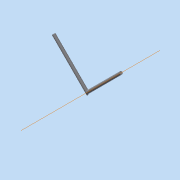
# Autodesk Inventor part: 00_Beampath_Autofocus
Saved by Autodesk Inventor 2019.4 (Build 234330000, 330)
## iProperties
Created: 2020-11-30
Part Number: 00_Beampath_Autofocus
Material: Generic
Document SubType Name: Modeling
Designer: diederichbenedict
Density: 1 g/cm^3
Appearance: Default
Author: diederichbenedict
Autodesk Inventor part; units mm, degrees
ref_plane "XY Plane" through (0, 0, 0) normal (0, 0, 1) x (1, 0, 0)
sketch "Sketch1" plane through (0, 0, 0) normal (0, 0, 1) x (1, 0, 0)
  line L0 (-5.1181, -14.425) -> (0.7509, -8.556) projected
  line L1 (-1.7947, -5.4447) -> (-0.1684, -7.0711) projected
  line L2 (0, 0) -> (12.9271, 0)
  line L3 (0, 0) -> (12.9271, 0) construction
  line L4 (-24, 24) -> (0, 0)
  line L5 (0, 0) -> (24, 24)
  line L6 (0, -22.11) -> (0, 31.685) projected
  dimension "d3" = 0
  dimension "d18" = 45
  dimension "d19" = 45
  dimension "d20" = 24
  dimension "d21" = 24
  constraints: 8 end point, 1 collinear, 1 horizontal
  measures "d3" distance between parallel lines of L2 L3
  measures "d18" angle of L6 L4
  measures "d19" angle of L5 L6
  measures "d20" horizontal distance of L2.start L4.start
  measures "d21" distance from line of L5.end L2
ref_plane "Work Plane3" through (0, 0, 0) normal (0.7071068, -0.7071068, 0) x (0, 0, -1)
sketch "Sketch5" plane through (0, 0, 0) normal (0.7071068, -0.7071068, 0) x (0, 0, -1)
  circle A0 centre (0, 0) radius 1
  dimension "d22" = 2
  constraints: 1 centre point, 1 coincident
  measures "d22" diameter of A0
sweep "Sweep2" add profiles "Sketch5" path "Sketch1" path curves L5 L4
sketch "Sketch6" plane through (0, 0, 0) normal (0, 1, 0) x (-1, 0, 0)
  ellipse E0 centre (0.2082, 1.8373) end of major axis (0.2082, 3.2873) minor radius 0.7088 (0.2082, 0.3873) -> (0.2082, 3.2873) ccw projected
  line L0 (0, -1) -> (0, 1) projected
  line L1 (0, 1) -> (0, -1) projected
  ellipse E1 centre (-24, 0) end of major axis (-24, 1) minor radius 0.7071 projected
  line L2 (-24, 1) -> (0, 1) projected
  line L3 (-24, -1) -> (0, -1) projected
  circle A0 centre (0, 0) radius 0.5
  dimension "d28" = 1
  dimension "d29" = 1
  constraints: 1 centre point, 1 coincident, 2 other
  measures "d28" diameter of A0
  measures "d29" distance from line of point (0, 0) L2
extrude "Extrusion3" add sketch "Sketch6" along normal mid plane 3 contours A0 L0 | L0 A0
body "Solid2"
